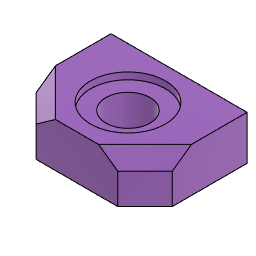
Z Linear Rail Endstop v5 (Autodesk Fusion 360 design; units mm, degrees)
Autodesk Fusion 360 part; units mm, degrees
sketch "Sketch1" plane through (0, 0, 0) normal (0, 0, 1) x (1, 0, 0)
  line L0 (10, 7.5) -> (-10, 7.5)
  line L1 (-10, 7.5) -> (-10, -7.5)
  line L2 (-10, -7.5) -> (10, -7.5)
  line L3 (10, -7.5) -> (10, 7.5)
  line L4 (10, 7.5) -> (-10, -7.5) construction
  line L5 (-10, 7.5) -> (10, -7.5) construction
  circle A0 centre (0, 0) radius 3.25
  dimension "d1" = 20
  dimension "d2" = 15
  dimension "d3" = 6.5
  constraint horizontal L0
  constraint perpendicular L0 L1
  constraint parallel L0 L2
  constraint parallel L1 L3
  constraint coincident L4 A0.centre
  constraint coincident L5 A0.centre
  constraint coincident A0.centre origin
  measures "d1" distance of L0.start L0.end
  measures "d2" distance of L0.start L2.end
  measures "d3" diameter of A0
extrude "Extrude1" add sketch "Sketch1" along normal blind 6.5
chamfer "Chamfer1" distance 4 distance2 4 2 edges at (-10, -7.5, 3.25) (10, -7.5, 3.25) measured on face at (-10, 2.5, 2.1667) measured on face at (-3.3333, -7.5, 4.3333)
chamfer "Chamfer2" distance 2 distance2 2 2 edges at (-8, -5.5, 6.5) (8, -5.5, 6.5) measured on face at (-7.3333, -6.1667, 2.1667) measured on face at (8.6667, -4.8333, 2.1667)
sketch "Sketch2" plane through (0, 0, 6.5) normal (0, 0, 1) x (-1, 0, 0)
  line L0 (-3.1716, 7.5) -> (-10, 0.6716)
  line L1 (-10, 0.6716) -> (-10, -7.5)
  line L2 (-10, -7.5) -> (10, -7.5)
  line L3 (10, -7.5) -> (10, 0.6716)
  line L4 (10, 0.6716) -> (3.1716, 7.5)
  line L5 (3.1716, 7.5) -> (-3.1716, 7.5)
  circle A0 centre (0, 0) radius 3.25
  circle A1 centre (0, 0) radius 5.5
  dimension "d10" = 11
  constraint concentric A0 A1
  measures "d10" diameter of A1
extrude "Extrude2" cut sketch "Sketch2" against normal blind 1 contours A1
